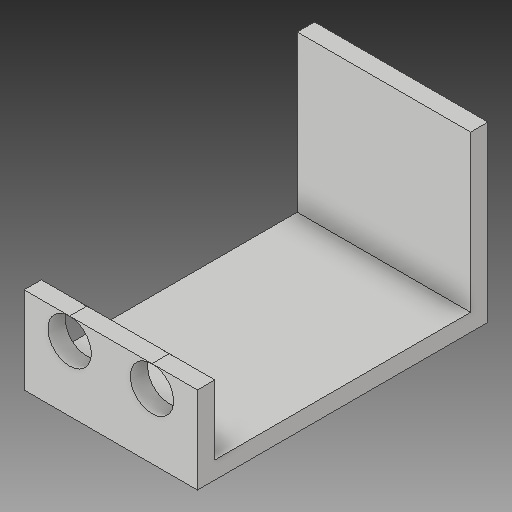
# Autodesk Inventor part: Servo Holder Bottom
Saved by Autodesk Inventor 2018 (Build 220112000, 112)
## iProperties
Created: 2018-04-21
Part Number: Servo Holder Bottom
Material: Generic
Document SubType Name: Modeling
Designer: HP
Density: 1 g/cm^3
Appearance: Default
Mass: 2.30146 g
Surface Area: 26.8229 cm^2
Volume: 2.30146 cm^3
Author: HP
Autodesk Inventor part; units mm, degrees
ref_plane "YZ Plane" through (0, 0, 0) normal (1, 0, 0) x (0, 1, 0)
ref_plane "XZ Plane" through (0, 0, 0) normal (0, 1, 0) x (-1, 0, 0)
ref_plane "XY Plane" through (0, 0, 0) normal (0, 0, 1) x (1, 0, 0)
sketch "Sketch1" plane through (0, 0, 0) normal (0, 1, 0) x (-1, 0, 0)
  line L0 (-20, 0) -> (0, 0)
  line L1 (0, 0) -> (0, -29.5)
  line L2 (0, -29.5) -> (-20, -29.5)
  line L3 (-20, -29.5) -> (-20, 0)
  dimension "d1" = 20
  dimension "d2" = 29.5
  constraints: 8 end point, 2 parallel, 1 horizontal, 1 perpendicular
  measures "d1" distance of L0.start L0.end
  measures "d2" distance of L2.end L0.start
sketch "Sketch2" plane through (0, 0, 0) normal (0, 0, 1) x (1, 0, 0)
  point P0 (0, 0)
extrude "Extrusion1" add sketch "Sketch1" along normal blind 2
sketch "Sketch3" plane through (0, 0, 0) normal (0, 0, 1) x (1, 0, 0)
  line L0 (20, 0) -> (0, 0) projected
  line L1 (0, 0) -> (20, 0)
  line L2 (20, 0) -> (20, 10)
  line L3 (20, 10) -> (0, 10)
  line L4 (0, 10) -> (0, 0)
  dimension "d11" = 10
  constraints: 8 end point, 2 parallel, 1 horizontal, 1 perpendicular
  measures "d11" distance of L2.end L1.end
extrude "Extrusion2" add sketch "Sketch3" along normal blind 2
sketch "Sketch4" plane through (0, 0, 2) normal (0, 0, 1) x (1, 0, 0)
  circle A0 centre (5.25, 7.5) radius 2.5
  circle A1 centre (14.75, 7.5) radius 2.5
  line L0 (20, 10) -> (0, 10) projected
  line L1 (0, 10) -> (0, 0) projected
  dimension "d18" = 5
  dimension "d19" = 5
  dimension "d20" = 2.5
  dimension "d21" = 2.5
  dimension "d22" = 9.5
  dimension "d23" = 5.25
  constraints: 2 centre point
  measures "d18" diameter of A0
  measures "d19" diameter of A1
  measures "d20" distance from line of L0 A0.centre
  measures "d21" distance from line of L0 A1.centre
  measures "d22" distance of A1.centre A0.centre
  measures "d23" distance from line of L1 A0.centre
extrude "Extrusion3" cut sketch "Sketch4" against normal blind 2 contours A1
sketch "Sketch5" plane through (0, 0, 2) normal (0, 0, 1) x (1, 0, 0)
  circle A0 centre (5.25, 7.5) radius 2.5
  line L0 (14.75, 10) -> (0, 10) projected
  circle A1 centre (14.75, 7.5) radius 2.5 projected
  point P0 (0, 0)
  dimension "d26" = 5
  dimension "d27" = 2.5
  dimension "d28" = 9.5
  constraints: 1 centre point, 1 vertical alignment
  measures "d26" diameter of A0
  measures "d27" distance from line of L0 A0.centre
  measures "d28" distance of point (14.75, 7.5) A0.centre
extrude "Extrusion4" cut sketch "Sketch5" against normal blind 2 contours A0
sketch "Sketch7" plane through (20, 0, -29.5) normal (0, 0, -1) x (-1, 0, 0)
  line L0 (20, 0) -> (0, 0) projected
  line L1 (0, 0) -> (20, 0)
  line L2 (20, 0) -> (20, 20)
  line L3 (20, 20) -> (0, 20)
  line L4 (0, 20) -> (0, 0)
  dimension "d34" = 20
  constraints: 8 end point, 2 parallel, 1 horizontal, 1 perpendicular
  measures "d34" distance of L2.end L1.end
extrude "Extrusion6" add sketch "Sketch7" along normal blind 2
body "Solid1"
